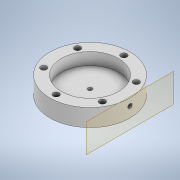
# Autodesk Inventor part: valve housing
Saved by Autodesk Inventor 2020 (Build 240168000, 168)
## iProperties
Created: 2020-08-08
Part Number: valve housing
Material: Generic
Document SubType Name: Modeling
Designer: benny
Density: 1 g/cm^3
Appearance: Default
Author: benny
Autodesk Inventor part; units mm, degrees
ref_plane "XZ Plane" through (0, 0, 0) normal (0, 1, 0) x (-1, 0, 0)
ref_plane "XY Plane" through (0, 0, 0) normal (0, 0, 1) x (1, 0, 0)
sketch "Sketch1" plane through (0, 0, 0) normal (0, 1, 0) x (-1, 0, 0)
  circle A0 centre (0, 0) radius 46
  dimension "d0" = 92
  constraints: 1 centre point, 1 coincident
  measures "d0" diameter of A0
extrude "Extrusion1" add sketch "Sketch1" along normal blind 20
sketch "Sketch2" plane through (0, 20, 0) normal (0, 1, 0) x (1, 0, 0)
  circle A0 centre (0, 0) radius 33
  dimension "d3" = 66
  constraints: 1 centre point, 1 coincident
  measures "d3" diameter of A0
extrude "Extrusion2" cut sketch "Sketch2" against normal blind 14
sketch "Sketch3" plane through (0, 6, 0) normal (0, 1, 0) x (1, 0, 0)
  circle A0 centre (0, 0) radius 2.5
  dimension "d6" = 5
  constraints: 1 centre point, 1 coincident
  measures "d6" diameter of A0
extrude "Extrusion3" cut sketch "Sketch3" against normal blind 6
sketch "Sketch4" plane through (0, 0, 0) normal (0, -1, 0) x (1, 0, 0)
  circle A0 centre (0, 0) radius 12
  dimension "d9" = 24
  constraints: 1 centre point, 1 coincident
  measures "d9" diameter of A0
extrude "Extrusion4" add sketch "Sketch4" along normal blind 10
sketch "Sketch5" plane through (0, 0, 0) normal (0, -1, 0) x (1, 0, 0)
  circle A0 centre (0, 0) radius 2.5 projected
  line L0 (0, 0) -> (0, -39)
  circle A1 centre (0, -39) radius 3.5
  dimension "d12" = 39
  dimension "d13" = 7
  constraints: 2 end point, 1 centre point, 1 coincident, 1 vertical
  measures "d12" distance of L0.start L0.end
  measures "d13" diameter of A1
extrude "Extrusion5" cut sketch "Sketch5" against normal blind 20 contours A1
pattern_circular "Circular Pattern1" count 6 over 360 about axis through (0, 0, 0) along (0, -1, 0) of "Extrusion5"
sketch "Sketch6" plane through (0, -10, 0) normal (0, -1, 0) x (1, 0, 0)
  circle A0 centre (0, 0) radius 2.5 projected
  circle A1 centre (0, 0) radius 7
  dimension "d19" = 14
  constraints: 1 centre point, 1 coincident
  measures "d19" diameter of A1
extrude "Extrusion6" cut sketch "Sketch6" against normal blind 10 contours A0 | A1
ref_plane "Work Plane2" through (46, 0, 0) normal (1, 0, 0) x (0, 1, 0)
sketch "Sketch8" plane through (46, 0, 0) normal (1, 0, 0) x (0, 1, 0)
  point P0 (0, 0)
  point P1 (12, 0)
  point P2 (12, 0)
  constraints: 1 coincident
hole "Hole1" at (46, 12, 0) direction (-1, 0, 0) diameter 4.917 depth 13 tip angle 118 thread size "M6x1" class "6H" standard "ISO Metric profile"
body "Solid1"
